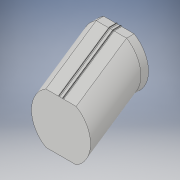
# Autodesk Inventor part: ramp top connect
Saved by Autodesk Inventor 2017 (Build 210142000, 142)
## iProperties
Created: 2018-03-06
Part Number: ramp top connect
Material: Generic
Document SubType Name: Modeling
Designer: braxtonwright
Density: 1 g/cm^3
Appearance: Default
Author: braxtonwright
Autodesk Inventor part; units mm, degrees
ref_plane "YZ Plane" through (0, 0, 0) normal (1, 0, 0) x (0, 1, 0)
ref_plane "XZ Plane" through (0, 0, 0) normal (0, 1, 0) x (-1, 0, 0)
ref_plane "XY Plane" through (0, 0, 0) normal (0, 0, 1) x (1, 0, 0)
sketch "Sketch1" plane through (0, 0, 0) normal (0, 0, 1) x (1, 0, 0)
  line L0 (-50.8, -84.6667) -> (50.8, -84.6667)
  arc A0 (-50.8, 84.6667) -> (-50.8, -84.6667) centre (0, 0) ccw
  arc A1 (50.8, -84.6667) -> (50.8, 84.6667) centre (0, 0) ccw
  line L1 (0, 84.67) -> (0, 87.8623) construction
  line L2 (-7.4083, 87.8623) -> (-7.4083, 86.2542)
  line L3 (7.4083, 87.8623) -> (7.4083, 86.2542)
  line L4 (8.9958, 84.6667) -> (50.8, 84.6667)
  line L5 (-8.9958, 84.6667) -> (8.9958, 84.6667) construction
  arc A2 (7.4083, 86.2542) -> (8.9958, 84.6667) centre (8.9958, 86.2542) ccw
  arc A3 (-8.9958, 84.6667) -> (-7.4083, 86.2542) centre (-8.9958, 86.2542) ccw
  line L6 (-8.9958, 84.6667) -> (-50.8, 84.6667)
  line L7 (0, 84.6667) -> (0, 87.8623) construction
  line L8 (6.35, 87.8623) -> (0, 87.8623) construction
  line L9 (6.3485, 84.6873) -> (3.1735, 87.8623) construction
  arc A4 (6.35, 87.8623) -> (3.1736, 84.6667) centre (6.3485, 84.6873) ccw construction
  arc A5 (4.1034, 84.6667) -> (6.35, 86.6385) centre (4.1034, 86.9324) ccw
  line L10 (6.35, 87.8623) -> (6.35, 86.6385)
  line L11 (-4.1034, 84.6667) -> (0, 84.6667)
  line L12 (-6.3485, 84.6873) -> (-3.1735, 87.8623) construction
  line L13 (-6.35, 87.8623) -> (-6.35, 86.6385)
  line L14 (-6.35, 87.8623) -> (0, 87.8623) construction
  arc A6 (-6.35, 86.6385) -> (-4.1034, 84.6667) centre (-4.1034, 86.9324) ccw
  arc A7 (-3.1736, 84.6667) -> (-6.35, 87.8623) centre (-6.3485, 84.6873) ccw construction
  line L15 (4.1034, 84.6667) -> (0, 84.6667)
  line L16 (7.4083, 87.8623) -> (6.35, 87.8623)
  line L17 (-6.35, 87.8623) -> (-7.4083, 87.8623)
  dimension "d66" = 101.6
  dimension "d67" = 14.8167
  dimension "d68" = 98.7374
  dimension "d69" = 98.7374
  dimension "d70" = 43.3917
  dimension "d71" = 1.5875
  dimension "d72" = 1.5875
  dimension "d73" = 41.8042
  dimension "d74" = 6.35
  dimension "d75" = 3.175
  dimension "d76" = 2.2657
  dimension "d77" = 2.2466
  dimension "d78" = 45
  dimension "d79" = 84.6667
  constraints: 36 end point, 19 point on circle, 10 symmetric about line, 8 centre point, 6 point on line, 4 collinear, 4 perpendicular, 3 coincident, 2 horizontal, 2 tangent, 1 parallel, 1 vertical, 4 other
  measures "d66" distance of L6.end L4.end
  measures "d67" distance of L2.start L3.start
  measures "d68" radius of A0
  measures "d69" radius of A1
  measures "d70" distance from line of L6.end L2
  measures "d71" distance from line of L4.start L3
  measures "d72" radius of A2
  measures "d73" distance of L4.start L4.end
  measures "d74" distance of L1.end L14.start
  measures "d75" distance of L14.start L12.start
  measures "d76" radius of A6
  measures "d77" horizontal distance of L11.start L13.end
  measures "d78" angle of L14 L12
  measures "d79" distance from line of L0 point (0, 0)
extrude "connecction top" add sketch "Sketch1" against normal blind 25.4
ref_plane "Work Plane2" through (0, 0, 203.2) normal (0, 0, 1) x (1, 0, 0)
sketch "Sketch6" plane through (0, 0, 0) normal (1, 0, 0) x (0, 1, 0)
  line L0 (-84.6667, 0) -> (-198.2947, 168.4604)
  line L1 (-84.6667, 0) -> (84.6667, 0) projected
  point P0 (0, 0)
  dimension "d28" = 203.2
  dimension "d65" = 124
  constraints: 2 end point
  measures "d28" distance of L0.start L0.end
  measures "d65" angle of L1 L0
sweep "ramp" add profiles "Sketch1" path "Sketch6" path curves L0
equation "\"d69\" = d68"
equation "\"d71\" = 0.5 * d80"
equation "\"d80\" = 3.175"
body "Solid1"
